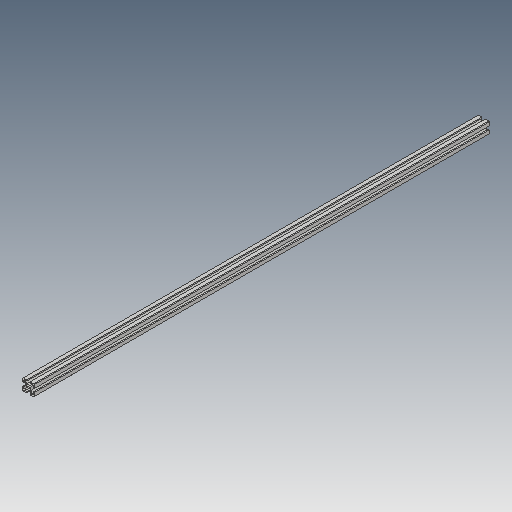
# Autodesk Inventor part: 高剛性フレーム
Saved by Autodesk Inventor 2020.3 (Build 243373000, 373)
## iProperties
Part Number: 高剛性フレーム
Material: 一般
Document SubType Name: Modeling
Designer: highs
Density: 1 g/cm^3
Appearance: 既定
Description: https://jp.misumi-ec.com/vona2/detail/110302683830/?HissuCode=HFS5-2020-800&PNSearch=HFS5-2020-800&KWSearch=HFS5-2020-800&searchFlow=results2products
Stock Number: HFS5-2020-800
Author: highs
Revision Number: 追加工なし
Autodesk Inventor part; units mm, degrees
ref_plane "YZ Plane" through (0, 0, 0) normal (1, 0, 0) x (0, 1, 0)
ref_plane "XZ Plane" through (0, 0, 0) normal (0, 1, 0) x (-1, 0, 0)
ref_plane "XY Plane" through (0, 0, 0) normal (0, 0, 1) x (1, 0, 0)
sketch "スケッチ1" plane through (0, 0, 0) normal (0, 0, 1) x (1, 0, 0)
  line L0 (-10, -10) -> (10, 10) construction
  line L1 (10, -10) -> (-10, 10) construction
  line L2 (10, 3) -> (8, 3)
  line L3 (8, 3) -> (8, 6.8686)
  line L4 (8, 6.8686) -> (4, 2.8686)
  line L5 (4, 2.8686) -> (4, -2.8686)
  line L6 (4, -2.8686) -> (8, -6.8686)
  line L7 (8, -6.8686) -> (8, -3)
  line L8 (8, -3) -> (10, -3)
  line L9 (-10, 0) -> (10, 0) construction
  line L10 (-3, 10) -> (-3, 8)
  line L11 (-3, 8) -> (-6.8686, 8)
  line L12 (-6.8686, 8) -> (-2.8686, 4)
  line L13 (-2.8686, 4) -> (2.8686, 4)
  line L14 (3, 8) -> (3, 10)
  line L15 (2.8686, 4) -> (6.8686, 8)
  line L16 (6.8686, 8) -> (3, 8)
  line L17 (-10, -3) -> (-8, -3)
  line L18 (-8, -3) -> (-8, -6.8686)
  line L19 (-8, -6.8686) -> (-4, -2.8686)
  line L20 (-4, -2.8686) -> (-4, 2.8686)
  line L21 (-8, 3) -> (-10, 3)
  line L22 (-4, 2.8686) -> (-8, 6.8686)
  line L23 (-8, 6.8686) -> (-8, 3)
  line L24 (3, -10) -> (3, -8)
  line L25 (3, -8) -> (6.8686, -8)
  line L26 (6.8686, -8) -> (2.8686, -4)
  line L27 (2.8686, -4) -> (-2.8686, -4)
  line L28 (-3, -8) -> (-3, -10)
  line L29 (-2.8686, -4) -> (-6.8686, -8)
  line L30 (-6.8686, -8) -> (-3, -8)
  line L31 (9, 10) -> (3, 10)
  line L32 (-3, 10) -> (-9, 10)
  line L33 (-10, 9) -> (-10, 3)
  line L34 (-10, -3) -> (-10, -9)
  line L35 (-9, -10) -> (-3, -10)
  line L36 (3, -10) -> (9, -10)
  line L37 (10, -9) -> (10, -3)
  line L38 (10, 3) -> (10, 9)
  circle A0 centre (0, 0) radius 2.1
  arc A1 (-9, 10) -> (-10, 9) centre (-9, 9) ccw
  arc A2 (-10, -9) -> (-9, -10) centre (-9, -9) ccw
  arc A3 (9, -10) -> (10, -9) centre (9, -9) ccw
  arc A4 (10, 9) -> (9, 10) centre (9, 9) ccw
  point P0 (0, 10)
  point P1 (-10, 0)
  point P2 (0, -10)
  dimension "d0" = 2
  dimension "d1" = 6
  dimension "d2" = 4
  dimension "d3" = 0.8
  dimension "d9" = 20
  dimension "d10" = 4.2
  dimension "d11" = 1
  constraints: 78 end point, 16 point on line, 10 parallel, 8 perpendicular, 8 point on circle, 8 tangent, 5 centre point, 3 equal radius, 3 horizontal, 2 midpoint, 1 coincident, 68 other
  measures "d0" distance of L7.end L8.end
  measures "d1" distance between parallel lines of L8 L2
  measures "d2" distance from line of L5 point (0, 0)
  measures "d3" distance between parallel lines of L0 L4
  measures "d9" distance between parallel lines of L36 L31
  measures "d10" diameter of A0
  measures "d11" radius of A1
extrude "押し出し1" add sketch "スケッチ1" along normal blind 800
